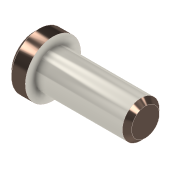
# Autodesk Inventor part: Axle
Saved by Autodesk Inventor 2022.2 (Build 262287010, 287A)
## iProperties
Created: 2022-12-29
Part Number: Axle
Material: Steel
Document SubType Name: Modeling
Designer: User
Mass: 1.4016 g
Surface Area: 2.10059 cm^2
Volume: 0.178547 cm^3
Density: 7.85 g/cm^3
Appearance: Gunmetal - Antique Polished
Author: User
Autodesk Inventor part; units mm, degrees
ref_plane "YZ Plane" through (0, 0, 0) normal (1, 0, 0) x (0, 1, 0)
ref_plane "XZ Plane" through (0, 0, 0) normal (0, 1, 0) x (-1, 0, 0)
ref_plane "XY Plane" through (0, 0, 0) normal (0, 0, 1) x (1, 0, 0)
sketch "Sketch1" plane through (0, 0, 0) normal (0, 0, 1) x (1, 0, 0)
  line L0 (0, 0) -> (0, 3)
  line L1 (0, 3) -> (2, 3)
  line L2 (2, 3) -> (2, 2)
  line L3 (2, 2) -> (12, 2)
  line L4 (12, 2) -> (12, 0)
  line L5 (12, 0) -> (0, 0)
  point P0 (1, 3)
  point P1 (0, 1.5)
  point P2 (2, 2.5)
  dimension "d0" = 6
  dimension "d1" = 4
  dimension "d2" = 12
  dimension "d3" = 2
  constraints: 12 end point, 3 midpoint, 3 perpendicular, 3 vertical, 1 coincident
  measures "d0" diameter of point (1, 3) L5
  measures "d1" diameter of L3 L5
  measures "d2" distance from line of L4 point (0, 1.5)
  measures "d3" distance from line of point (2, 2.5) L0
revolve "Revolution1" add sketch "Sketch1" angle 360 about axis through (12, 0, 0) along (-1, 0, 0)
chamfer "Chamfer1" distance 0.5 angle 45 2 edges at (0, -3, 0) (12, -2, 0)
body "Solid1"
